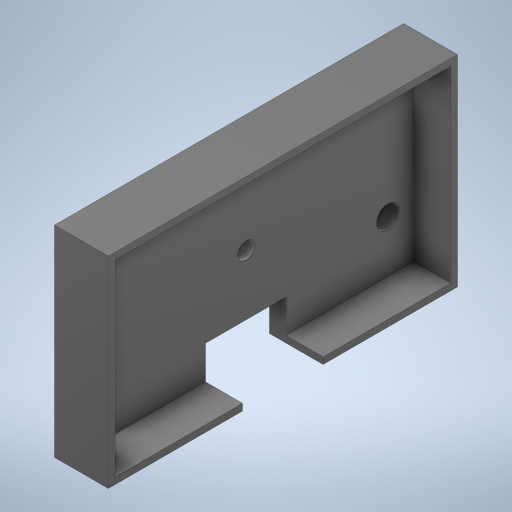
# Autodesk Inventor part: SensorHalter
Saved by Autodesk Inventor 2023 (Build 270158000, 158)
## iProperties
Created: 2024-01-25
Part Number: SensorHalter
Material: Generisch
Document SubType Name: Modeling
Designer: phili
Density: 1 g/cm^3
Appearance: Vorgabe
Author: phili
Autodesk Inventor part; units mm, degrees
ref_plane "YZ Plane" through (0, 0, 0) normal (1, 0, 0) x (0, 1, 0)
ref_plane "XZ Plane" through (0, 0, 0) normal (0, 1, 0) x (-1, 0, 0)
ref_plane "XY Plane" through (0, 0, 0) normal (0, 0, 1) x (1, 0, 0)
sketch "Skizze1" plane through (0, 0, 0) normal (1, 0, 0) x (0, 1, 0)
  line L0 (-15, -26) -> (15, -26)
  line L1 (15, -26) -> (15, 26)
  line L2 (15, 26) -> (-15, 26)
  line L3 (-15, 26) -> (-15, -26)
  line L4 (-15, -26) -> (15, 26) construction
  line L5 (15, -26) -> (-15, 26) construction
  point P0 (0, 0)
  dimension "d0" = 30
  dimension "d1" = 52
  constraints: 12 end point, 2 midpoint, 2 parallel, 1 horizontal, 1 perpendicular
  measures "d0" distance of L2.end L1.end
  measures "d1" distance of L1.end L0.end
extrude "Extrusion1" add sketch "Skizze1" along normal blind 8
sketch "Skizze2" plane through (8, 0, 0) normal (1, 0, 0) x (0, 0, -1)
  line L0 (25, -14) -> (-25, -14)
  line L1 (-25, -14) -> (-25, 14)
  line L2 (-25, 14) -> (25, 14)
  line L3 (25, 14) -> (25, -14)
  line L4 (25, -14) -> (-25, 14) construction
  line L5 (-25, -14) -> (25, 14) construction
  point P0 (0, 0)
  dimension "d4" = 50
  dimension "d5" = 28
  constraints: 12 end point, 2 midpoint, 2 parallel, 1 horizontal, 1 perpendicular
  measures "d4" distance of L1.end L2.end
  measures "d5" distance of L0.end L1.end
extrude "Extrusion2" cut sketch "Skizze2" against normal blind 5.5
sketch "Skizze3" plane through (2.5, 0, 0) normal (1, 0, 0) x (0, 0, -1)
  line L0 (-26, -15) -> (26, -15) projected
  line L1 (-6, -15) -> (6, -15)
  line L2 (6, -15) -> (6, -9)
  line L3 (6, -9) -> (-6, -9)
  line L4 (-6, -9) -> (-6, -15)
  point P0 (0, 0)
  point P1 (6, -15)
  dimension "d8" = 12
  dimension "d9" = 6
  dimension "d10" = 6
  constraints: 8 end point, 2 parallel, 1 horizontal, 1 perpendicular, 1 point on line
  measures "d8" distance of L3.end L2.end
  measures "d9" distance of L2.end L1.end
  measures "d10" distance from line of L4 point (0, 0)
extrude "Extrusion3" cut sketch "Skizze3" along normal through all both and the other way through all
sketch "Skizze4" plane through (2.5, 0, 0) normal (1, 0, 0) x (0, 0, -1)
  point P0 (0, 0)
  point P1 (-21.125, 11)
  point P2 (21.125, 11)
  point P3 (21.125, -6.25)
  point P4 (-21.125, -6.25)
  dimension "d20" = 17.25
  dimension "d21" = 17.25
  dimension "d22" = 11
  dimension "d23" = 11
  dimension "d24" = 42.25
  dimension "d25" = 42.25
  dimension "d26" = 21.125
  dimension "d27" = 21.125
  measures "d20" distance of point (-21.125, -6.25) point (-21.125, 11)
  measures "d21" distance of point (21.125, -6.25) point (21.125, 11)
  measures "d22" vertical distance of point (0, 0) point (-21.125, 11)
  measures "d23" vertical distance of point (0, 0) point (21.125, 11)
  measures "d24" distance of point (21.125, 11) point (-21.125, 11)
  measures "d25" distance of point (21.125, -6.25) point (-21.125, -6.25)
  measures "d26" horizontal distance of point (0, 0) point (-21.125, 11)
  measures "d27" horizontal distance of point (0, 0) point (-21.125, -6.25)
hole "Bohrung1" at (2.5, 11, 21.125) at (2.5, 11, -21.125) at (2.5, -6.25, -21.125) at (2.5, -6.25, 21.125) direction (-1, 0, 0) diameter 3.4 end through all
sketch "Skizze7" plane through (2.5, 0, 0) normal (1, 0, 0) x (0, 0, -1)
  point P0 (0, 0)
  point P1 (0, 0)
  dimension "d51" = 0
  dimension "d52" = 0
  measures "d51" distance of point (0, 0) point (0, 0)
  measures "d52" distance of point (0, 0) point (0, 0)
hole "Bohrung3" at (2.5, 0, 0) direction (-1, 0, 0) diameter 2.5 end through all
